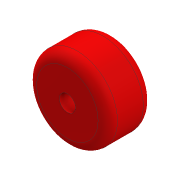
# Autodesk Inventor part: castor_wheel
Saved by Autodesk Inventor 2020 (Build 240168000, 168)
## iProperties
Created: 2020-09-08
Part Number: castor_wheel
Material: 고무, 실리콘
Document SubType Name: Modeling
Designer: 이호석
Mass: 7.88778 g
Surface Area: 20.5168 cm^2
Volume: 6.31022 cm^3
Density: 1.25 g/cm^3
Appearance: 고무 - 검은색
Author: 이호석
Autodesk Inventor part; units mm, degrees
ref_plane "YZ Plane" through (0, 0, 0) normal (1, 0, 0) x (0, 1, 0)
ref_plane "XZ Plane" through (0, 0, 0) normal (0, 1, 0) x (-1, 0, 0)
ref_plane "XY Plane" through (0, 0, 0) normal (0, 0, 1) x (1, 0, 0)
sketch "스케치1" plane through (0, 0, 0) normal (0, 0, 1) x (1, 0, 0)
  circle A0 centre (0, 0) radius 12.5
  circle A1 centre (0, 0) radius 2.5
  dimension "d0" = 25
  dimension "d1" = 5
  constraints: 2 centre point, 2 coincident
  measures "d0" diameter of A0
  measures "d1" diameter of A1
extrude "돌출1" add sketch "스케치1" along normal blind 14
fillet "모깎기1" radius 3 2 edges at (-12.5, 0, 14) (-12.5, 0, 0)
